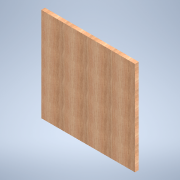
# Autodesk Inventor part: Table
Saved by Autodesk Inventor 2022 (Build 260153000, 153)
## iProperties
Created: 2022-03-19
Part Number: Table
Material: Wood (Birch)
Document SubType Name: Modeling
Designer: dvorakj
Density: 0.55 g/cm^3
Appearance: Birch - Natural Polished
Author: dvorakj
Autodesk Inventor part; units mm, degrees
ref_plane "YZ Plane" through (0, 0, 0) normal (1, 0, 0) x (0, 1, 0)
ref_plane "XZ Plane" through (0, 0, 0) normal (0, 1, 0) x (-1, 0, 0)
ref_plane "XY Plane" through (0, 0, 0) normal (0, 0, 1) x (1, 0, 0)
sketch "Sketch1" plane through (0, 0, 0) normal (0, 0, 1) x (1, 0, 0)
  line L0 (0, 0) -> (-1000, 0)
  line L1 (-1000, 0) -> (-1000, -1000)
  line L2 (-1000, -1000) -> (0, -1000)
  line L3 (0, -1000) -> (0, 0)
  dimension "d0" = 1000
  dimension "d1" = 1000
  constraints: 8 end point, 2 parallel, 1 horizontal, 1 perpendicular
  measures "d0" distance of L2.end L1.end
  measures "d1" distance of L1.end L0.end
extrude "Extrusion1" add sketch "Sketch1" along normal blind 40
body "Solid1"
